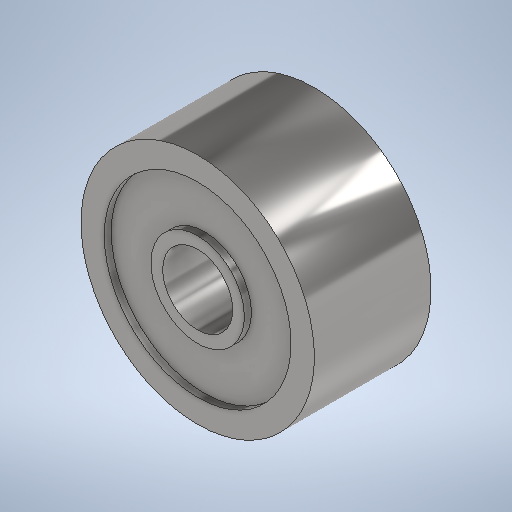
# Autodesk Inventor part: Bearing_BS69310-5
Saved by Autodesk Inventor 2025.1 (Build 291241020, 241B)
## iProperties
Created: 2024-11-07
Part Number: Bearing_BS69310-5
Material: Generic
Document SubType Name: Modeling
Designer: leon-
Density: 1 g/cm^3
Appearance: Steel - Polished
Author: leon-
Autodesk Inventor part; units mm, degrees
ref_plane "YZ Plane" through (0, 0, 0) normal (1, 0, 0) x (0, 1, 0)
ref_plane "XZ Plane" through (0, 0, 0) normal (0, 1, 0) x (-1, 0, 0)
ref_plane "XY Plane" through (0, 0, 0) normal (0, 0, 1) x (1, 0, 0)
sketch "Sketch1" plane through (0, 0, 0) normal (1, 0, 0) x (0, 1, 0)
  line L0 (5, 0) -> (1.5, 0)
  line L1 (1.5, 0) -> (1.5, -2.5)
  line L2 (5, -2.5) -> (5, 0)
  line L3 (-1, 0) -> (6, 0) projected
  line L4 (0, -3) -> (0, 0.5) projected
  line L5 (1.5, -2.5) -> (2, -2.5)
  line L6 (2, -2.5) -> (2, -2.2)
  line L7 (2, -2.2) -> (4, -2.2)
  line L8 (4, -2.2) -> (4, -2.5)
  line L9 (4, -2.5) -> (5, -2.5)
  point P0 (0, 0)
  point P1 (4, -2.35)
  point P2 (2, -2.35)
  dimension "d1" = 5
  dimension "d2" = 1.5
  dimension "d5" = 2.2
  dimension "d6" = 1
  dimension "d7" = 0.5
  dimension "d9" = 2.5
  constraints: 16 end point, 5 perpendicular, 2 horizontal, 2 midpoint, 1 collinear, 1 parallel, 1 point on line
  measures "d1" distance from line of point (0, 0) L2
  measures "d2" distance from line of point (0, 0) L1
  measures "d5" distance between parallel lines of L3 L7
  measures "d6" distance from line of point (4, -2.35) L2
  measures "d7" distance from line of point (2, -2.35) L1
  measures "d9" distance between parallel lines of L3 L9
revolve "Revolution1" add sketch "Sketch1" angle 360 about axis through (0, 0, -10) along (0, 0, 1)
mirror "Mirror1" about plane through (0, 0, 0) normal (0, 0, 1) of "Revolution1"
body "Solid1"
